Battery Holder July 13 (Autodesk Fusion 360 design; units mm, degrees)
Autodesk Fusion 360 part; units mm, degrees
note: some values were not read from the file. Set by a fixed rule: which sketch regions a step uses.
sketch "Sketch1" plane through (0, 0, 0) normal (0, 0, 1) x (1, 0, 0)
  line L0 (36.1, 25.85) -> (-36.1, 25.85)
  line L1 (-36.1, 25.85) -> (-36.1, -25.85)
  line L2 (-36.1, -25.85) -> (36.1, -25.85)
  line L3 (36.1, -25.85) -> (36.1, 25.85)
  line L4 (36.1, 25.85) -> (-36.1, -25.85) construction
  line L5 (-36.1, 25.85) -> (36.1, -25.85) construction
  line L6 (-39.1, 28.85) -> (-39.1, -28.85)
  line L7 (-39.1, -28.85) -> (39.1, -28.85)
  line L8 (39.1, -28.85) -> (39.1, 28.85)
  line L9 (39.1, 28.85) -> (-39.1, 28.85)
  dimension "d1" = 72.2
  dimension "d2" = 51.7
  dimension "d3" = 3
  measures "d1" distance of L1 L3
  measures "d2" distance of L0 L2
extrude "Extrude1" add sketch "Sketch1" along normal blind 20 makes body 1
extrude "Extrude2" add sketch "Sketch1" against normal blind 2 contours L0 L1 L2 L3 | L6 L7 L8 L9 bodies 1
sketch "Sketch2" plane through (0, 0, 0) normal (0, 0, 1) x (1, 0, 0)
  line L0 (36.1, 25.85) -> (-36.1, 25.85)
  line L1 (-36.1, 25.85) -> (-36.1, -25.85)
  line L2 (-36.1, -25.85) -> (36.1, -25.85)
  line L3 (36.1, -25.85) -> (36.1, 25.85)
  line L4 (21, 17) -> (-21, 17)
  line L5 (-25, 13) -> (-25, -13)
  line L6 (-21, -17) -> (21, -17)
  line L7 (25, -13) -> (25, 13)
  line L8 (25, 17) -> (-25, -17) construction
  line L9 (-25, 17) -> (25, -17) construction
  arc A0 (-25, -13) -> (-21, -17) centre (-21, -13) ccw
  arc A1 (-21, 17) -> (-25, 13) centre (-21, 13) ccw
  arc A2 (25, 13) -> (21, 17) centre (21, 13) ccw
  arc A3 (21, -17) -> (25, -13) centre (21, -13) ccw
  dimension "d8" = 34
  dimension "d9" = 50
  dimension "d10" = 4
  dimension "d11" = 4
  dimension "d12" = 4
  dimension "d13" = 4
  measures "d8" distance of L8.start L9.end
  measures "d9" distance of L5 L7
  measures "d10" radius of A0
  measures "d11" radius of A1
  measures "d12" radius of A2
  measures "d13" radius of A3
extrude "Extrude3" cut sketch "Sketch2" against normal blind 5 contours L4 L5 L6 L7 A0 A1 A2 A3 bodies 1
fillet "Fillet1" radius 4 4 edges at (-39.1, -28.85, 9) (-39.1, 28.85, 9) (39.1, 28.85, 9) (39.1, -28.85, 9) on bodies 1
fillet "Fillet2" radius 2 4 edges at (-36.1, 25.85, 10) (36.1, 25.85, 10) (36.1, -25.85, 10) (-36.1, -25.85, 10) on bodies 1
ref_plane "WorkPlane1" through (0, 0, 9) normal (1, 0, 0) x (0, 1, 0)
sketch "Sketch3" plane through (0, 0, 3) normal (1, 0, 0) x (0, 0, -1)
  line L0 (5, 28.85) -> (-17, 28.85)
  line L1 (-17, 28.85) -> (5, 28.85)
  line L2 (-16, 28.85) -> (-6, 30.85)
  line L3 (-6, 30.85) -> (-6, 28.85)
  dimension "d18" = 1
  dimension "d19" = 2
  measures "d18" distance of L0.end L2.start
  measures "d19" distance of L2.end L3.end
extrude "Extrude4" add sketch "Sketch3" along normal mid plane 30 bodies 1
ref_plane "WorkPlane2" through (0, 0, 9) normal (0, -1, 0) x (1, 0, 0)
mirror "Mirror1" about plane through (0, 0, 9) normal (0, -1, 0) of "Extrude4"
ref_plane "WorkPlane3" through (0, 0, 9) normal (0, -1, 0) x (1, 0, 0)
sketch "Sketch4" plane through (39.1, 0, 0) normal (1, 0, 0) x (0, 0, -1)
  line L0 (-20, -24.85) -> (2, -24.85)
  line L1 (2, -24.85) -> (2, 24.85)
  line L2 (2, 24.85) -> (-20, 24.85)
  line L3 (-20, 24.85) -> (-20, -24.85)
  line L4 (-20, -10) -> (2, -10)
  line L5 (2, -10) -> (2, -14)
  line L6 (2, -14) -> (-20, -14)
  line L7 (-20, -14) -> (-20, -10)
  line L8 (2, 0) -> (-20, 0) construction
  line L9 (-20, 10) -> (2, 10)
  line L10 (2, 14) -> (-20, 14)
  dimension "d23" = 4
  dimension "d24" = 10
  measures "d23" distance of L4 L6
  measures "d24" distance of origin L4
extrude "Extrude5" add sketch "Sketch4" along normal blind 1 contours L1 L3 L4 L5 L6 L7 | L1 L3 L9 L10 bodies 1
ref_plane "WorkPlane4" through (0, 0, 9) normal (1, 0, 0) x (0, 1, 0)
mirror "Mirror2" about plane through (0, 0, 9) normal (1, 0, 0) of "Extrude5"
fillet "Fillet3" radius 2 2 edges at (0, 28.85, 9) (0, -28.85, 9) on bodies 1
extrude "Extrude6" add 1 faces at (-7, -24.9, -2) along direction (0, 0, -1) blind 2 on bodies 1 bodies 1
ref_plane "WorkPlane5" through (0, 0, 30) normal (0, 0, 1) x (1, 0, 0)
sketch "Sketch5" plane through (0, 0, 30) normal (0, 0, 1) x (1, 0, 0)
  arc A0 (35.1, -28.85) -> (39.1, -24.85) centre (35.1, -24.85) ccw
  line L0 (39.1, -24.85) -> (39.1, -14)
  line L1 (39.1, -14) -> (40.1, -14)
  line L2 (40.1, -14) -> (40.1, -10)
  line L3 (40.1, -10) -> (39.1, -10)
  line L4 (39.1, -10) -> (39.1, 10)
  line L5 (39.1, 10) -> (40.1, 10)
  line L6 (40.1, 10) -> (40.1, 14)
  line L7 (40.1, 14) -> (39.1, 14)
  line L8 (39.1, 14) -> (39.1, 24.85)
  arc A1 (39.1, 24.85) -> (35.1, 28.85) centre (35.1, 24.85) ccw
  line L9 (35.1, 28.85) -> (-35.1, 28.85)
  arc A2 (-35.1, 28.85) -> (-39.1, 24.85) centre (-35.1, 24.85) ccw
  line L10 (-39.1, 24.85) -> (-39.1, 14)
  line L11 (-39.1, 14) -> (-40.1, 14)
  line L12 (-40.1, 14) -> (-40.1, 10)
  line L13 (-40.1, 10) -> (-39.1, 10)
  line L14 (-39.1, 10) -> (-39.1, -10)
  line L15 (-39.1, -10) -> (-40.1, -10)
  line L16 (-40.1, -10) -> (-40.1, -14)
  line L17 (-40.1, -14) -> (-39.1, -14)
  line L18 (-39.1, -14) -> (-39.1, -24.85)
  arc A3 (-39.1, -24.85) -> (-35.1, -28.85) centre (-35.1, -24.85) ccw
  line L19 (-35.1, -28.85) -> (35.1, -28.85)
  line L20 (36.1, 23.85) -> (36.1, -23.85)
  arc A4 (34.1, -25.85) -> (36.1, -23.85) centre (34.1, -23.85) ccw
  line L21 (34.1, -25.85) -> (-34.1, -25.85)
  arc A5 (-36.1, -23.85) -> (-34.1, -25.85) centre (-34.1, -23.85) ccw
  line L22 (-36.1, -23.85) -> (-36.1, 23.85)
  arc A6 (-34.1, 25.85) -> (-36.1, 23.85) centre (-34.1, 23.85) ccw
  line L23 (-34.1, 25.85) -> (34.1, 25.85)
  arc A7 (36.1, 23.85) -> (34.1, 25.85) centre (34.1, 23.85) ccw
extrude "Extrude7" add sketch "Sketch5" along normal blind 2 separate body contours A0 L0 L1 L2 L3 L4 L5 L6 L7 L8 A1 L9 A2 L10 L11 L12 L13 L14 L15 L16 L17 L18 A3 L19 | L20 A4 L21 A5 L22 A6 L23 A7 makes body 2
extrude "Extrude8" add sketch "Sketch5" against normal blind 9.75 bodies 2
sketch "Sketch6" plane through (39.1, 0, 0) normal (1, 0, 0) x (0, 0, -1)
  line L0 (-20.25, 10) -> (-32, 10)
  line L1 (-32, 10) -> (-32, -10)
  line L2 (-32, -10) -> (-20.25, -10)
  line L3 (-20.25, -10) -> (-20.25, 10)
  line L4 (-32, 10) -> (-20.25, 10)
  line L5 (-20.25, 10) -> (-20.25, -10)
  line L6 (-20.25, -10) -> (-32, -10)
  line L7 (-32, -10) -> (-32, 10)
extrude "Extrude9" add sketch "Sketch6" along normal blind 2 bodies 2
sketch "Sketch7" plane through (0, 0, 20.25) normal (0, 0, -1) x (-1, 0, 0)
  arc A0 (-36.1, -23.85) -> (-34.1, -25.85) centre (-34.1, -23.85) ccw
  line L0 (-36.1, -23.85) -> (-36.1, 23.85)
  arc A1 (-34.1, 25.85) -> (-36.1, 23.85) centre (-34.1, 23.85) ccw
  line L1 (-34.1, 25.85) -> (34.1, 25.85)
  arc A2 (36.1, 23.85) -> (34.1, 25.85) centre (34.1, 23.85) ccw
  line L2 (36.1, 23.85) -> (36.1, -23.85)
  arc A3 (34.1, -25.85) -> (36.1, -23.85) centre (34.1, -23.85) ccw
  line L3 (34.1, -25.85) -> (-34.1, -25.85)
  line L4 (-35.1, -28.85) -> (35.1, -28.85)
  arc A4 (35.1, -28.85) -> (39.1, -24.85) centre (35.1, -24.85) ccw
  line L5 (39.1, -24.85) -> (39.1, -14)
  line L6 (39.1, -14) -> (40.1, -14)
  line L7 (40.1, -14) -> (40.1, -10)
  line L8 (40.1, -10) -> (39.1, -10)
  line L9 (39.1, -10) -> (39.1, 10)
  line L10 (39.1, 10) -> (40.1, 10)
  line L11 (40.1, 10) -> (40.1, 14)
  line L12 (40.1, 14) -> (39.1, 14)
  line L13 (39.1, 14) -> (39.1, 24.85)
  arc A5 (39.1, 24.85) -> (35.1, 28.85) centre (35.1, 24.85) ccw
  line L14 (35.1, 28.85) -> (-35.1, 28.85)
  arc A6 (-35.1, 28.85) -> (-39.1, 24.85) centre (-35.1, 24.85) ccw
  line L15 (-39.1, 24.85) -> (-39.1, 14)
  line L16 (-39.1, 14) -> (-40.1, 14)
  line L17 (-40.1, 14) -> (-40.1, 10)
  line L18 (-40.1, 10) -> (-41.1, 10)
  line L19 (-41.1, 10) -> (-41.1, -10)
  line L20 (-41.1, -10) -> (-40.1, -10)
  line L21 (-40.1, -10) -> (-40.1, -14)
  line L22 (-40.1, -14) -> (-39.1, -14)
  line L23 (-39.1, -14) -> (-39.1, -24.85)
  arc A7 (-39.1, -24.85) -> (-35.1, -28.85) centre (-35.1, -24.85) ccw
  line L24 (-41.1, -9.7) -> (-39.4, -9.7)
  line L25 (-39.4, -9.7) -> (-39.4, 9.7)
  line L26 (-39.4, 9.7) -> (-41.1, 9.7)
  line L27 (-41.1, 9.7) -> (-41.1, -9.7)
  line L28 (-39.1, 10) -> (-39.1, -10)
  dimension "d38" = 0.3
  dimension "d39" = 0.3
  dimension "d40" = 0.3
  measures "d38" distance of L18 L26
  measures "d39" distance of L20.end L24
  measures "d40" distance of L25 L28
extrude "Extrude10" add sketch "Sketch7" along normal blind 10 contours L19 L24 L25 L26 L27 bodies 2
mirror "Mirror3" about plane through (0, 0, 9) normal (1, 0, 0) of "Extrude9", "Extrude10"
sketch "Sketch8" plane through (0, -28.85, 0) normal (0, -1, 0) x (1, 0, 0)
  line L0 (35.1, 20.25) -> (35.1, 32)
  line L1 (35.1, 32) -> (-35.1, 32)
  line L2 (-35.1, 32) -> (-35.1, 20.25)
  line L3 (-35.1, 20.25) -> (35.1, 20.25)
  line L4 (-25.1, 31) -> (25.1, 31)
  line L5 (25.1, 31) -> (25.1, 29)
  line L6 (25.1, 29) -> (-25.1, 29)
  line L7 (-25.1, 29) -> (-25.1, 31)
  dimension "d44" = 10
  dimension "d45" = 10
  dimension "d46" = 1
  dimension "d47" = 2
  measures "d44" distance of L2 L7
  measures "d45" distance of L0 L5
  measures "d46" distance of L1 L4
  measures "d47" distance of L4 L6
extrude "Extrude11" add sketch "Sketch8" along normal blind 1.8 contours L4 L5 L6 L7 bodies 2
sketch "Sketch9" plane through (25.1, 0, 0) normal (1, 0, 0) x (0, 0, -1)
  line L0 (-29, -28.85) -> (-31, -28.85)
  line L1 (-31, -28.85) -> (-31, -30.65)
  line L2 (-31, -30.65) -> (-29, -30.65)
  line L3 (-29, -30.65) -> (-29, -28.85)
  line L4 (-31, -30.65) -> (-7, -30.65)
  line L5 (-7, -30.65) -> (-7, -32.65)
  line L6 (-7, -32.65) -> (-31, -32.65)
  line L7 (-31, -32.65) -> (-31, -30.65)
  circle A0 centre (-8, -30.65) radius 1
  line L8 (-20.25, -30.65) -> (-22.25, -30.65)
  line L9 (-22.25, -30.65) -> (-22.25, -29.05)
  line L10 (-22.25, -29.05) -> (-20.25, -29.05)
  line L11 (-20.25, -29.05) -> (-20.25, -30.65)
  line L12 (-20.25, -28.85) -> (-20.25, -24.85)
  line L13 (-32, -28.85) -> (-20.25, -28.85)
  point P0 (-9, -30.85)
  dimension "d50" = 2
  dimension "d51" = 2
  dimension "d52" = 2
  dimension "d55" = 2
  dimension "d56" = 0.2
  measures "d50" distance of L4 L6
  measures "d51" distance of L5 P0
  measures "d52" diameter of A0
  measures "d55" distance of L9 L11
  measures "d56" distance of L10 L13
extrude "Extrude12" add sketch "Sketch9" against normal up to surface (50.2 mm away) separate body contours L2 L4 L5 L6 L7 A0 L8 | L4 L8 L9 L10 L11 | L4 A0 | L4 A0 makes body 3
mirror "Mirror4" about plane through (0, 0, 0) normal (0, 1, 0) of bodies 3 makes body 4
mirror "Mirror5" about plane through (0, 0, 0) normal (0, 1, 0) of "Extrude11"
combine "Combine1" operation add target body 2 tool bodies 4 3
fillet "Fillet4" radius 2 4 edges at (0, 30.65, 29) (0, 32.65, 31) (0, -32.65, 31) (0, -30.65, 29) on bodies 2
sketch "Sketch10" plane through (-39.1, 0, 0) normal (-1, 0, 0) x (0, 0, 1)
  line L0 (20, -14) -> (-4, -14)
  line L1 (-4, -14) -> (-4, -24.85)
  line L2 (-4, -24.85) -> (20, -24.85)
  line L3 (20, -24.85) -> (20, -14)
  line L4 (20, -16.925) -> (12, -16.925)
  line L5 (10, -18.925) -> (10, -19.925)
  line L6 (12, -21.925) -> (20, -21.925)
  line L7 (20, -21.925) -> (20, -16.925)
  arc A0 (10, -19.925) -> (12, -21.925) centre (12, -19.925) ccw
  arc A1 (12, -16.925) -> (10, -18.925) centre (12, -18.925) ccw
  point P0 (20, -19.425)
  point P1 (20, -19.425)
  dimension "d60" = 10
  dimension "d61" = 5
  dimension "d62" = 2
  dimension "d63" = 2
  measures "d60" distance of L5 L7
  measures "d61" distance of L4 L6
  measures "d62" radius of A0
  measures "d63" radius of A1
extrude "Extrude13" cut sketch "Sketch10" against normal blind 4 contours L3 L4 L5 L6 L7 A0 A1 bodies 1
sketch "Sketch11" plane through (0, 0, 32) normal (0, 0, 1) x (1, 0, 0)
  line L0 (-35.1, -28.85) -> (35.1, -28.85)
  arc A0 (35.1, -28.85) -> (39.1, -24.85) centre (35.1, -24.85) ccw
  line L1 (39.1, -24.85) -> (39.1, -14)
  line L2 (39.1, -14) -> (40.1, -14)
  line L3 (40.1, -14) -> (40.1, -10)
  line L4 (40.1, -10) -> (41.1, -10)
  line L5 (41.1, -10) -> (41.1, 10)
  line L6 (41.1, 10) -> (40.1, 10)
  line L7 (40.1, 10) -> (40.1, 14)
  line L8 (40.1, 14) -> (39.1, 14)
  line L9 (39.1, 14) -> (39.1, 24.85)
  arc A1 (39.1, 24.85) -> (35.1, 28.85) centre (35.1, 24.85) ccw
  line L10 (35.1, 28.85) -> (-35.1, 28.85)
  arc A2 (-35.1, 28.85) -> (-39.1, 24.85) centre (-35.1, 24.85) ccw
  line L11 (-39.1, 24.85) -> (-39.1, 14)
  line L12 (-39.1, 14) -> (-40.1, 14)
  line L13 (-40.1, 14) -> (-40.1, 10)
  line L14 (-40.1, 10) -> (-41.1, 10)
  line L15 (-41.1, 10) -> (-41.1, -10)
  line L16 (-41.1, -10) -> (-40.1, -10)
  line L17 (-40.1, -10) -> (-40.1, -14)
  line L18 (-40.1, -14) -> (-39.1, -14)
  line L19 (-39.1, -14) -> (-39.1, -24.85)
  arc A3 (-39.1, -24.85) -> (-35.1, -28.85) centre (-35.1, -24.85) ccw
  line L20 (25, -13) -> (25, 13)
  line L21 (21, 17) -> (-21, 17)
  arc A4 (25, 13) -> (21, 17) centre (21, 13) ccw
  arc A5 (21, -17) -> (25, -13) centre (21, -13) ccw
  line L22 (-21, -17) -> (21, -17)
  arc A6 (-25, -13) -> (-21, -17) centre (-21, -13) ccw
  line L23 (-25, 13) -> (-25, -13)
  arc A7 (-21, 17) -> (-25, 13) centre (-21, 13) ccw
  point P0 (21, -17)
  point P1 (25, -13)
extrude "Extrude14" cut sketch "Sketch11" against normal blind 10 contours L20 L21 A4 A5 L22 A6 L23 A7 bodies 2
sketch "Sketch12" plane through (25, 0, 0) normal (-1, 0, 0) x (0, 0, 1)
  line L0 (-4, -13) -> (0, -13)
  line L1 (0, -13) -> (0, 13)
  line L2 (0, 13) -> (-4, 13)
  line L3 (-4, 13) -> (-4, -13)
  line L4 (-4, 3.85) -> (-6, 3.85)
  line L5 (-6, 3.85) -> (-6, -3.85)
  line L6 (-6, -3.85) -> (-4, -3.85)
  line L7 (-4, -3.85) -> (-4, 3.85)
  line L8 (-4, 7.5) -> (0, 7.5)
  line L9 (0, 7.5) -> (0, -7.5)
  line L10 (0, -7.5) -> (-4, -7.5)
  line L11 (-4, -7.5) -> (-4, 7.5)
  point P0 (-4, 0)
  dimension "d68" = 7.7
  dimension "d69" = 2
  dimension "d70" = 15
  measures "d68" distance of L4.end L5.end
  measures "d69" distance of L5.end L6.end
  measures "d70" distance of L8 L10
extrude "Extrude15" add sketch "Sketch12" against normal blind 30 contours L1 L3 L7 L8 L9 L10 L11 | L3 L4 L5 L6 L7 L11 bodies 1
sketch "Sketch13" plane through (0, 0, 0) normal (0, 0, 1) x (1, 0, 0)
  line L0 (39.1, 7.5) -> (39.1, -7.5)
  line L1 (39.1, -7.5) -> (55, -7.5)
  line L2 (55, -7.5) -> (55, 7.5)
  line L3 (55, 7.5) -> (39.1, 7.5)
  circle A0 centre (48, 0) radius 3.2
  point P0 (55, 0)
  dimension "d73" = 6.4
  dimension "d74" = 7
  measures "d73" diameter of A0
  measures "d74" distance of L2 A0.centre
extrude "Extrude16" cut sketch "Sketch13" against normal blind 7 contours A0 bodies 1
mirror "Mirror6" about plane through (0, 0, 0) normal (1, 0, 0) of "Extrude15", "Extrude16"
equation "d39 = d38"
equation "d40 = d38"
